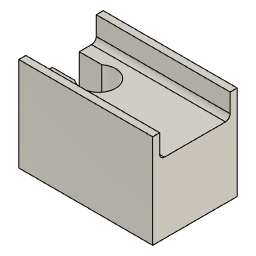
BTT Filament Sensor Pedestal (Autodesk Fusion 360 design; units mm, degrees)
Autodesk Fusion 360 part; units mm, degrees
sketch "Sketch1" plane through (0, 0, 0) normal (0, 0, 1) x (1, 0, 0)
  line L0 (28.5, -18) -> (-28.5, -18)
  line L1 (-28.5, -18) -> (-28.5, 18)
  line L2 (-28.5, 18) -> (28.5, 18)
  line L3 (28.5, 18) -> (28.5, -18)
  line L4 (28.5, -18) -> (-28.5, 18) construction
  line L5 (-28.5, -18) -> (28.5, 18) construction
  dimension "d1" = 57
  dimension "d2" = 36
  constraint horizontal L0
  constraint perpendicular L0 L1
  constraint parallel L0 L2
  constraint parallel L1 L3
  constraint coincident L4 origin
  constraint coincident L5 origin
  measures "d1" distance of L0.start L0.end
  measures "d2" distance of L0.start L2.end
extrude "Extrude1" add sketch "Sketch1" along normal blind 30
sketch "Sketch2" plane through (0, 0, 30) normal (0, 0, 1) x (-1, 0, 0)
  line L0 (-28.5, -18) -> (28.5, -18)
  line L1 (28.5, -18) -> (28.5, 18)
  line L2 (28.5, 18) -> (-28.5, 18)
  line L3 (-28.5, 18) -> (-28.5, -18)
  line L4 (28.5, 18) -> (28.5, 15)
  line L5 (-28.5, 15) -> (28.5, 15)
  line L6 (-28.5, 15) -> (-28.5, 18)
  line L7 (-28.5, 18) -> (28.5, 18)
  dimension "d7" = 3
  constraint coincident L1.end L2.start
  constraint coincident L1 L4.end
  constraint perpendicular L2 L4
  constraint coincident L3 L5.start
  constraint perpendicular L3 L5
  constraint coincident L2.end L3.start
  constraint perpendicular L2 L6
  measures "d7" distance of L5.start L2.end
extrude "Extrude2" add sketch "Sketch2" along normal blind 10 contours L1 L2 L3 L4 L5 L6 L7
mirror "Mirror1" about plane through (0, 0, 0) normal (0, 1, 0) of "Extrude2"
sketch "Sketch3" plane through (0, 0, 30) normal (0, 0, 1) x (-1, 0, 0)
  line L0 (-28.5, -15) -> (28.5, -15)
  line L1 (28.5, -15) -> (28.5, 15)
  line L2 (28.5, 15) -> (-28.5, 15)
  line L3 (-28.5, 15) -> (-28.5, -15)
  circle A0 centre (14.5, -2) radius 7.25
  dimension "d10" = 14.5
  dimension "d11" = 14
  dimension "d15" = 17
  dimension "d18" = 13
  measures "d10" diameter of A0
  measures "d11" distance of L1 A0.centre
  measures "d15" distance of L2 A0.centre
  measures "d18" distance of L0 A0.centre
extrude "Extrude3" cut sketch "Sketch3" against normal through all contours A0
sketch "Sketch4" plane through (0, 0, 30) normal (0, 0, 1) x (-1, 0, 0)
  circle A0 centre (14.5, -2) radius 7.25
  line L0 (-28.5, -15) -> (28.5, -15)
  line L1 (28.5, -15) -> (28.5, 15)
  line L2 (28.5, 15) -> (-28.5, 15)
  line L3 (-28.5, 15) -> (-28.5, -15)
  line L4 (18.9159, -7.75) -> (28.5, -7.75)
  line L5 (28.5, -7.75) -> (28.5, 3.75)
  line L6 (18.9159, 3.75) -> (18.9159, -7.75)
  line L7 (18.9159, 3.75) -> (28.5, 3.75)
  dimension "d13" = 11.5
  constraint coincident A0 L4.start
  constraint coincident L1 L4.end
  constraint perpendicular L1 L4
  constraint coincident L1 L5.end
  constraint coincident A0 L6.start
  constraint vertical L6
  constraint horizontal L7
  measures "d13" distance of L4.end L5.end
extrude "Extrude4" cut sketch "Sketch4" against normal through all contours A0 L1 L4 L5 L7
fillet "Fillet1" radius 2 2 edges at (0, -15, 30) (0, 15, 30)
